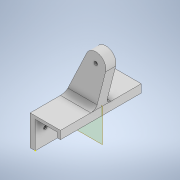
# Autodesk Inventor part: holder
Saved by Autodesk Inventor 2020 (Build 240168000, 168)
## iProperties
Created: 2022-10-15
Part Number: holder
Material: Типовые
Document SubType Name: Modeling
Designer: zigma
Density: 1 g/cm^3
Appearance: По умолчанию
Author: zigma
Autodesk Inventor part; units mm, degrees
ref_plane "YZ Plane" through (0, 0, 0) normal (1, 0, 0) x (0, 1, 0)
ref_plane "XZ Plane" through (0, 0, 0) normal (0, 1, 0) x (-1, 0, 0)
ref_plane "XY Plane" through (0, 0, 0) normal (0, 0, 1) x (1, 0, 0)
sketch "Эскиз1" plane through (0, 0, 0) normal (0, 0, 1) x (1, 0, 0)
  line L0 (30, 30) -> (0, 30)
  line L1 (0, 30) -> (0, 0)
  line L2 (30, 30) -> (30, 22)
  line L3 (5, 0) -> (5, 27)
  line L4 (5, 27) -> (27, 27)
  line L5 (27, 27) -> (27, 22)
  line L6 (0, 0) -> (5, 0)
  line L7 (27, 22) -> (30, 22)
  dimension "d0" = 30
  dimension "d2" = 30
  dimension "d5" = 5
  dimension "d6" = 8
  dimension "d15" = 3
  dimension "d16" = 3
  dimension "d17" = 5
  constraints: 16 end point, 1 horizontal, 1 parallel, 1 vertical
  measures "d0" distance of L0.end L0.start
  measures "d2" distance of L0.end L1.end
  measures "d5" distance of L4.end L5.end
  measures "d6" distance of L0.start L2.end
  measures "d15" distance between parallel lines of L4 L0
  measures "d16" distance between parallel lines of L5 L2
  measures "d17" distance between parallel lines of L1 L3
extrude "Выдавливание1" add sketch "Эскиз1" against normal blind 80
sketch "Эскиз2" plane through (0, 0, 0) normal (-1, 0, 0) x (0, 0, 1)
  line L0 (0, 30) -> (-80, 30) projected
  line L1 (-70, 30) -> (-70, 0) construction
  line L2 (0, 0) -> (-80, 0) projected
  circle A0 centre (-70, 15) radius 3 construction
  line L3 (-68.2679, 18) -> (-66.5359, 15)
  line L4 (-66.5359, 15) -> (-68.2679, 12)
  line L5 (-68.2679, 12) -> (-71.7321, 12)
  line L6 (-71.7321, 12) -> (-73.4641, 15)
  line L7 (-73.4641, 15) -> (-71.7321, 18)
  line L8 (-71.7321, 18) -> (-68.2679, 18)
  line L9 (-80, 0) -> (-80, 30) projected
  line L10 (0, 30) -> (-80, 30) projected
  point P0 (-70, 18)
  dimension "d9" = 6
  dimension "d30" = 10
  constraints: 14 end point, 2 midpoint, 1 coincident, 1 point on line, 1 vertical alignment, 15 other
  measures "d30" distance between parallel lines of L9 L1
extrude "Выдавливание2" cut sketch "Эскиз2" against normal blind 4
sketch "Эскиз3" plane through (4, 0, 0) normal (-1, 0, 0) x (0, 0, 1)
  line L0 (-71.7321, 18) -> (-68.2679, 18) projected
  line L1 (-70, 18) -> (-70, 12) construction
  line L2 (-68.2679, 12) -> (-71.7321, 12) projected
  circle A0 centre (-70, 15) radius 1.75
  point P0 (0, 0)
  dimension "d18" = 3.5
  constraints: 3 midpoint, 2 end point, 1 centre point
  measures "d18" diameter of A0
extrude "Выдавливание3" cut sketch "Эскиз3" against normal up to next
ref_plane "РабПлоскость1" through (0, 0, -40) normal (0, 0, -1) x (-1, 0, 0)
sketch "Эскиз4" plane through (0, 0, -40) normal (0, 0, -1) x (-1, 0, 0)
  arc A0 (-20.9616, 74.2788) -> (-39.6825, 67.5) centre (-30, 70) ccw
  line L0 (-30, 30) -> (-30, 22) projected
  line L1 (-30, 30) -> (-39.6825, 67.5)
  line L2 (0, 30) -> (0, 0) projected
  line L3 (0, 30) -> (-20.9616, 74.2788)
  circle A1 centre (-30, 70) radius 1.75
  line L4 (-30, 22) -> (-30, 30)
  line L5 (-30, 30) -> (0, 30)
  line L6 (-30, 22) -> (-27, 22) projected
  dimension "d21" = 20
  dimension "d22" = 3.5
  dimension "d31" = 30
  dimension "d32" = 40
  constraints: 8 end point, 2 centre point, 2 point on circle, 2 tangent, 1 coincident, 1 perpendicular, 1 vertical
  measures "d21" diameter of A0
  measures "d22" diameter of A1
  measures "d31" distance from line of L2 A0.centre
  measures "d32" distance from line of A0.centre L5
extrude "Выдавливание4" add sketch "Эскиз4" along normal mid plane 10
fillet "Сопряжение1" radius 5 2 edges at (15, 30, -45) (15, 30, -35)
mirror "Зеркальное отражение1" about plane through (0, 0, -40) normal (0, 0, -1) of "Выдавливание2", "Выдавливание3"
sketch "Эскиз5" plane through (5, 0, 0) normal (1, 0, 0) x (0, 0, -1)
  point P0 (0, 0)
equation "\"d6\" = d5 + d4"
equation "\"d4\" = 3"
